Autodesk Fusion 360 part; units mm, degrees
(part 3 of 3)
extrude "Extrude24" cut sketch "front/back_ribSlots" against normal blind 463.55 contours L0 L6 L7 L8 L10 | L0 L6 L8 L9 L10 | L0 L25 L27 L28 | L0 L25 L26 L27 bodies 2
extrude "Extrude25" add sketch "top_ribSlots" along normal mid plane 12.7 separate body contours L0 L3 L73 | L0 L3 L74 L75 L76 L77 L78 L79 L80 L81 L82 L83 L84 L85 | L1 L2 L7 L61 L62 L63 L64 L65 L66 L67 L68 L69 L70 L71 L72 | L1 L2 L7 L60 | L2 L3 L6 L59 | L2 L3 L6 L39 L40 L41 L42 L45 L46 L47 L48 L49 L53 | L0 L1 L8 L86 | L0 L1 L8 L87 L88 L89 L90 L91 L92 L93 L94 L95 L96 L97 L98 | L41 L53 L54 L55 L56 | L42 L49 L50 L51 L52 makes body 9 at (-469.9, 6.35, -428.625) makes body 10 at (469.9, 6.35, -428.625) makes body 11 at (-469.9, 6.35, 428.625) makes body 12 at (466.725, 6.35, 431.8)
extrude "Extrude26" add sketch "front/back_ribSlots" along normal blind 222.25 and the other way blind -209.55 separate body contours L0 L3 L6 L49 | L0 L3 L6 L50 L51 L52 L53 L54 L55 L56 L57 L58 L59 L60 L61 | L0 L1 L47 | L0 L1 L29 L30 L31 L32 L35 L36 L37 L38 L39 L43 | L31 L39 L40 L41 L42 | L32 L43 L44 L45 L46 makes body 13 at (466.725, 241.3, 209.55) makes body 14 at (-466.725, 241.3, 209.55)
extrude "Extrude27" add sketch "front/back_ribSlots" along normal blind -209.55 and the other way blind 222.25 separate body contours L0 L3 L6 L49 | L0 L3 L6 L50 L51 L52 L53 L54 L55 L56 L57 L58 L59 L60 L61 | L0 L1 L47 | L0 L1 L29 L30 L31 L32 L35 L36 L37 L38 L39 L43 | L31 L39 L40 L41 L42 | L32 L43 L44 L45 L46 makes body 15 at (-466.725, 241.3, -222.25) makes body 16 at (466.725, 241.3, -222.25)
extrude "Extrude28" add sketch "LR_ribSlots" along normal blind 241.3 and the other way blind -228.6 separate body contours L0 L3 L47 | L0 L3 L29 L30 L31 L32 L35 L36 L37 L38 L39 L43 | L31 L43 L44 L45 L46 | L32 L39 L40 L41 L42 makes body 17
extrude "Extrude29" add sketch "LR_ribSlots" along normal blind -228.6 and the other way blind 241.3 separate body contours L0 L3 L47 | L0 L3 L29 L30 L31 L32 L35 L36 L37 L38 L39 L43 | L31 L43 L44 L45 L46 | L32 L39 L40 L41 L42 makes body 18
extrude "Extrude30" add sketch "LR_ribSlots" along normal blind 425.45 and the other way blind -412.75 separate body contours L0 L1 L18 L49 | L0 L1 L18 L50 L51 L52 L53 L54 L55 L56 L57 L58 L59 L60 L61 makes body 19
extrude "Extrude31" add sketch "LR_ribSlots" along normal blind -412.75 and the other way blind 425.45 separate body contours L0 L1 L18 L49 | L0 L1 L18 L50 L51 L52 L53 L54 L55 L56 L57 L58 L59 L60 L61 makes body 20
hidden bodies 1
equation "enclosure_width = 39 in"
equation "enclosure_height = 21 in"
equation "enclosure_depth = 36 in"
equation "d4 = enclosure_width"
equation "d5 = enclosure_depth"
equation "d6 = enclosure_height"
equation "segment_width = 2 in"
equation "d10 = -segment_width"
equation "segment_thickness = 0.25 in"
equation "d49 = enclosure_width"
equation "d50 = enclosure_height"
equation "d51 = enclosure_width - ( segment_width * 2 )"
equation "d52 = enclosure_height - ( segment_width * 2 )"
equation "d65 = -enclosure_depth / 2"
equation "d67 = enclosure_depth / 2 + segment_thickness"
equation "d81 = enclosure_depth"
equation "d82 = enclosure_height"
equation "d83 = enclosure_depth - ( segment_width * 2 )"
equation "d84 = enclosure_height - ( segment_width * 2 )"
equation "d85 = enclosure_width / 2 + segment_thickness"
equation "d87 = -enclosure_width / 2"
equation "d89 = -enclosure_width / 2 - segment_thickness"
equation "d91 = enclosure_width / 2"
equation "d97 = enclosure_height / 2 + segment_thickness"
equation "d99 = -enclosure_height / 2"
equation "door_width = 27 in"
equation "door_height = 15 in"
equation "d109 = enclosure_depth / 2 + segment_thickness"
equation "d111 = -enclosure_depth / 2"
equation "door_depth = 16 in"
equation "d122 = enclosure_height / 2 + segment_thickness"
equation "d124 = -enclosure_height / 2"
equation "d127 = enclosure_depth / 2 + segment_thickness"
equation "d129 = -enclosure_depth / 2"
equation "segment_length = 17 in"
equation "doorFrame_segments = ( ceil(( door_depth - segment_width ) / segment_length) + 1 ) + ( ( ceil(( door_depth - segment_width ) / segment_length) + 1 ) % 2 )"
equation "door_depthSegments = ( ceil(( -door_depth + segment_width * 3 ) / segment_length) + 1 ) + ( ( ceil(( -door_depth + segment_width * 3 ) / segment_length) + 1 ) % 2 )"
equation "enclosureDepth_segments = ( ceil(( enclosure_depth - segment_width * 2 ) / segment_length) + 1 ) + ( ( ceil(( enclosure_depth - segment_width * 2 ) / segment_length) + 1 ) % 2 )"
equation "enclosureWidth_segments = ( ceil(( abs(enclosure_width - segment_width * 3) ) / segment_length) + 1 ) + ( ( ceil(( abs(enclosure_width - segment_width * 3) ) / segment_length) + 1 ) % 2 )"
equation "tolerance = 0.25 in"
equation "d202 = segment_width"
equation "d203 = segment_width"
equation "d204 = segment_width"
equation "d205 = segment_width"
equation "d206 = segment_width"
equation "d207 = segment_width"
equation "d208 = segment_width"
equation "d209 = segment_width"
equation "d210 = segment_width"
equation "d211 = segment_width"
equation "d212 = segment_width - ( 0.5 in + tolerance )"
equation "d213 = segment_width - ( 0.5 in + tolerance )"
equation "d214 = enclosureDepth_segments"
equation "d216 = enclosure_depth - segment_width * 2 - segment_width"
equation "d218 = segment_width"
equation "d219 = segment_width"
equation "d220 = segment_width"
equation "d221 = segment_width"
equation "d222 = segment_width - ( 0.5 in + tolerance )"
equation "d224 = segment_width - ( 0.5 in + tolerance )"
equation "d225 = segment_width - ( 0.5 in + tolerance )"
equation "d226 = segment_width"
equation "d227 = segment_width"
equation "d229 = segment_width - ( 0.5 in + tolerance )"
equation "d230 = segment_width - ( 0.5 in + tolerance )"
equation "d231 = segment_width - ( 0.5 in + tolerance )"
equation "enclosureHeight_segments = ( ceil(( enclosure_height - segment_width * 2 ) / segment_length) + 1 ) + ( ( ceil(( enclosure_height - segment_width * 2 ) / segment_length) + 1 ) % 2 )"
equation "d238 = enclosureHeight_segments"
equation "d240 = -enclosure_height + segment_width * 3"
equation "ribSlot_width = 0.5 in"
equation "ribSlot_height = 1.25 in"
equation "d259 = segment_width"
equation "d260 = segment_width"
equation "d261 = segment_width"
equation "d262 = segment_width"
equation "d263 = segment_width"
equation "d264 = segment_width"
equation "d265 = segment_width"
equation "d266 = segment_width"
equation "d267 = segment_width"
equation "d268 = segment_width"
equation "d269 = segment_width"
equation "d270 = segment_width"
equation "d271 = segment_width"
equation "d272 = segment_width"
equation "d273 = segment_width"
equation "d274 = segment_width"
equation "d275 = segment_width - ( 0.5 in + tolerance )"
equation "d276 = segment_width - ( 0.5 in + tolerance )"
equation "d277 = segment_width - ( 0.5 in + tolerance )"
equation "d278 = segment_width - ( 0.5 in + tolerance )"
equation "d279 = segment_width - ( 0.5 in + tolerance )"
equation "d280 = segment_width - ( 0.5 in + tolerance )"
equation "d281 = segment_width - ( 0.5 in + tolerance )"
equation "d282 = segment_width - ( 0.5 in + tolerance )"
equation "d283 = enclosureWidth_segments"
equation "d285 = enclosure_width - segment_width * 2 - segment_width"
equation "d296 = enclosureHeight_segments"
equation "d298 = -enclosure_height + segment_width * 2 + segment_width"
equation "door_widthSegments = ( ceil(( door_width - segment_width * 3 ) / segment_length) + 1 ) + ( ( ceil(( door_width - segment_width * 3 ) / segment_length) + 1 ) % 2 )"
equation "door_heightSegments = ( ceil(( abs(-door_height + segment_width * 2) ) / segment_length) + 1 ) + ( ( ceil(( abs(-door_height + segment_width * 2) ) / segment_length) + 1 ) % 2 )"
equation "frontLR_segments = ( ceil(( -door_height + segment_width * 2 ) / segment_length) + 1 ) + ( ( ceil(( -door_height + segment_width * 2 ) / segment_length) + 1 ) % 2 )"
equation "topBridge_segments = ( ceil(( door_width - segment_width ) / segment_length) + 1 ) + ( ( ceil(( door_width - segment_width ) / segment_length) + 1 ) % 2 )"
equation "frontB_segments = ( ( ( ceil(( enclosure_width - segment_width * 7 ) / segment_length) ) * 1 in + 1 in ) + ( ( ( ceil(( enclosure_width - segment_width * 7 ) / segment_length) + 1 ) % 2 ) * 1 in ) ) / in"
equation "topLR_segments = ( ceil(( abs(-enclosure_depth) - door_depth - segment_width * 2.5 ) / segment_length) + 1 ) + ( ( ceil(( abs(-enclosure_depth) - door_depth - segment_width * 2.5 ) / segment_length) + 1 ) % 2 )"
equation "d614 = enclosure_width"
equation "d615 = enclosure_depth"
equation "d616 = ( enclosure_width - door_width ) / 2"
equation "d617 = door_depth"
equation "d618 = ( enclosure_width - door_width ) / 2"
equation "d619 = door_depth"
equation "d620 = segment_width"
equation "d621 = segment_width"
equation "d622 = segment_width"
equation "d623 = segment_width"
equation "d624 = segment_width"
equation "d625 = segment_width"
equation "d626 = segment_width"
equation "d627 = segment_width"
equation "d628 = segment_width"
equation "d629 = segment_width"
equation "d630 = segment_width"
equation "d631 = segment_width"
equation "d632 = segment_width"
equation "d633 = segment_width"
equation "d634 = segment_width - ( 0.5 in + tolerance )"
equation "d635 = segment_width - ( 0.5 in + tolerance )"
equation "d637 = door_depthSegments"
equation "d639 = door_depth - segment_width * 3"
equation "d640 = segment_width"
equation "d641 = segment_width"
equation "d642 = segment_width - ( 0.5 in + tolerance )"
equation "d643 = segment_width - ( 0.5 in + tolerance )"
equation "d644 = door_widthSegments"
equation "d646 = door_width - segment_width * 3"
equation "d648 = segment_width"
equation "d649 = segment_width - ( 0.5 in + tolerance )"
equation "d650 = enclosureWidth_segments"
equation "d652 = enclosure_width - segment_width * 3"
equation "d654 = segment_width"
equation "d655 = segment_width - ( 0.5 in + tolerance )"
equation "d656 = segment_width"
equation "d657 = segment_width - ( 0.5 in + tolerance )"
equation "d659 = topLR_segments"
equation "d661 = -enclosure_depth + door_depth + segment_width * 3"
equation "d662 = segment_width"
equation "d663 = segment_width - ( 0.5 in + tolerance )"
equation "d665 = doorFrame_segments"
equation "d667 = -door_depth + segment_width * 2"
equation "d668 = segment_width"
equation "d669 = segment_width"
equation "d670 = segment_width"
equation "d671 = segment_width"
equation "d672 = segment_width"
equation "d673 = segment_width"
equation "d674 = segment_width - ( 0.5 in + tolerance )"
equation "d675 = segment_width - ( 0.5 in + tolerance )"
equation "d676 = segment_width - ( 0.5 in + tolerance )"
equation "d678 = doorFrame_segments"
equation "d680 = -door_depth + segment_width * 2"
equation "d681 = segment_width"
equation "d682 = segment_width"
equation "d683 = segment_width - ( 0.5 in + tolerance )"
equation "d684 = topBridge_segments"
equation "d686 = door_width - segment_width"
equation "d688 = enclosure_depth - segment_width"
equation "d689 = enclosure_height - segment_width"
equation "d690 = ribSlot_height"
equation "d691 = ribSlot_width"
equation "d692 = ribSlot_height"
equation "d693 = ribSlot_width"
equation "d694 = ( enclosure_depth - segment_width ) / 4"
equation "d695 = ribSlot_width"
equation "d696 = ribSlot_height"
equation "d699 = ( enclosure_depth - segment_width ) / 2"
equation "d701 = enclosure_width / 2 + segment_thickness"
equation "d703 = enclosure_width - segment_width"
equation "d704 = enclosure_depth - segment_width"
equation "d705 = ( enclosure_depth - segment_width ) / 4"
equation "d706 = ( enclosure_depth - segment_width ) / 4"
equation "d707 = ( enclosure_width - segment_width ) / 4"
equation "d708 = ribSlot_width"
equation "d709 = ribSlot_height"
equation "d710 = ribSlot_height"
equation "d711 = ribSlot_width"
equation "d712 = ribSlot_height"
equation "d713 = ribSlot_width"
equation "d717 = ( enclosure_depth - segment_width ) / 2"
equation "d720 = ( enclosure_width - segment_width ) / 2"
equation "d722 = enclosure_height / 2 + segment_thickness"
equation "d724 = enclosure_width - segment_width"
equation "d725 = enclosure_height - segment_width"
equation "d726 = ( enclosure_width - segment_width ) / 4"
equation "d727 = ribSlot_width"
equation "d728 = ribSlot_height"
equation "d729 = ribSlot_height"
equation "d730 = ribSlot_width"
equation "d731 = ribSlot_height"
equation "d732 = ribSlot_width"
equation "d735 = ( -enclosure_width + segment_width ) / 2"
equation "d737 = enclosure_depth / 2 + segment_thickness"
equation "d739 = -enclosure_depth / 2 - segment_thickness"
equation "d745 = ribSlot_width"
equation "d746 = ribSlot_height"
equation "d747 = ribSlot_width"
equation "d748 = ribSlot_height"
equation "d749 = segment_width"
equation "d750 = segment_width"
equation "d751 = ( segment_width - ribSlot_height ) / 2"
equation "d752 = ( segment_width - ribSlot_height ) / 2"
equation "d753 = ( segment_width - ribSlot_height ) / 2"
equation "d754 = ( segment_width - ribSlot_height ) / 2"
equation "d755 = segment_thickness"
equation "d756 = segment_thickness"
equation "d757 = segment_width / 2"
equation "d758 = d757"
equation "d759 = ribSlot_width / 2"
equation "d761 = segment_width"
equation "d762 = segment_width"
equation "d763 = ( segment_width - ribSlot_height ) / 2"
equation "d764 = ( segment_width - ribSlot_height ) / 2"
equation "d765 = ( segment_width - ribSlot_height ) / 2"
equation "d766 = ( segment_width - ribSlot_height ) / 2"
equation "d767 = segment_thickness"
equation "d768 = segment_thickness"
equation "d769 = segment_width / 2"
equation "d770 = d769"
equation "d771 = ( enclosure_depth / 2 - segment_width / 2 ) / 2 + ribSlot_width / 2"
equation "d773 = ( -enclosure_depth / 2 + segment_width / 2 ) / 2 + ribSlot_width / 2"
equation "d775 = ( -enclosure_depth / 2 + segment_width / 2 ) / 2 + ribSlot_width / 2"
equation "d777 = ( enclosure_depth / 2 - segment_width / 2 ) / 2 + ribSlot_width / 2"
equation "d779 = segment_width"
equation "d780 = segment_width"
equation "d782 = ( segment_width - ribSlot_height ) / 2"
equation "d783 = ( segment_width - ribSlot_height ) / 2"
equation "d784 = ( segment_width - ribSlot_height ) / 2"
equation "d785 = segment_thickness"
equation "d786 = segment_thickness"
equation "d787 = segment_width / 2"
equation "d788 = d787"
equation "d789 = ( enclosure_width / 2 - segment_width / 2 ) / 2 + ribSlot_width / 2"
equation "d791 = ( -enclosure_width / 2 + segment_width / 2 ) / 2 + ribSlot_width / 2"
equation "d793 = ( -enclosure_width / 2 + segment_width / 2 ) / 2 + ribSlot_width / 2"
equation "d795 = ( enclosure_width / 2 - segment_width / 2 ) / 2 + ribSlot_width / 2"
equation "d797 = door_width / 2 + ( enclosure_width - door_width ) / 4 + ribSlot_width / 2"
equation "d799 = -door_width / 2 - ( enclosure_width - door_width ) / 4 + ribSlot_width / 2"
equation "d801 = -door_width / 2 - ( enclosure_width - door_width ) / 4 + ribSlot_width / 2"
equation "d803 = door_width / 2 + ( enclosure_width - door_width ) / 4 + ribSlot_width / 2"
equation "d805 = enclosure_width"
equation "d806 = enclosure_height"
equation "d807 = ( enclosure_width - door_width ) / 2"
equation "d808 = segment_width"
equation "d809 = ( enclosure_width - door_width ) / 2"
equation "d810 = segment_width"
equation "d811 = door_height"
equation "d812 = segment_width"
equation "d813 = segment_width"
equation "d814 = segment_width"
equation "d815 = segment_width"
equation "d816 = segment_width"
equation "d817 = segment_width"
equation "d818 = segment_width"
equation "d819 = segment_width"
equation "d820 = segment_width"
equation "d821 = enclosure_height - door_height"
equation "d822 = enclosure_width"
equation "d823 = segment_width"
equation "d824 = segment_width"
equation "d825 = jointDiameter"
equation "d826 = enclosureWidth_segments"
equation "d828 = enclosure_width - segment_width * 3"
equation "jointDiameter = segment_width - ( 0.5 in + tolerance )"
equation "d831 = segment_width"
equation "d832 = jointDiameter"
equation "d833 = segment_width"
equation "d834 = jointDiameter"
equation "d835 = door_widthSegments"
equation "d837 = door_width - segment_width * 3"
equation "d839 = segment_width"
equation "d840 = segment_width"
equation "d841 = jointDiameter"
equation "d842 = jointDiameter"
equation "d844 = door_heightSegments"
equation "d846 = -door_height + segment_width * 3"
equation "d847 = segment_width"
equation "d848 = segment_width"
equation "d849 = segment_width"
equation "d850 = segment_width"
equation "d851 = jointDiameter"
equation "d852 = jointDiameter"
equation "d853 = jointDiameter"
equation "d854 = jointDiameter"
equation "d856 = doorFrame_segments"
equation "d858 = -door_height + segment_width * 2"
equation "d859 = segment_width"
equation "d860 = segment_width"
equation "d861 = jointDiameter"
equation "d862 = jointDiameter"
equation "d863 = ( enclosure_width - door_width ) / 2"
equation "d864 = segment_width"
equation "d865 = segment_width"
equation "d866 = jointDiameter"
equation "d867 = topBridge_segments"
equation "d869 = -door_width + segment_width"
equation "d871 = ribSlot_width"
equation "d872 = ribSlot_height"
equation "d873 = ribSlot_width"
equation "d874 = ribSlot_height"
named bodies: "machine_footprint", "frame_back", "frame_right", "frame_left", "frame_top", "frame_front", "accessDoor_front", "accessDoor_top", "backLeft_rib", "backRight_rib", "frontLeft_rib", "frontRight_rib", "topFrontRight_rib", "topFrontLeft_rib", "topBackLeft_rib", "topBackRight_rib", "backTopRight_rib", "backTopLeft_rib", "frontTopRight_rib", "frontTopLeft_rib"
